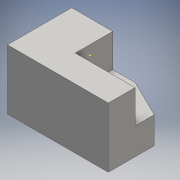
# Autodesk Inventor part: 240503_3Dsketch04
Saved by Autodesk Inventor 2016 (Build 200138000, 138)
## iProperties
Created: 2024-05-03
Part Number: 240503_3Dsketch04
Material: 일반
Document SubType Name: Modeling
Designer: pc
Density: 1 g/cm^3
Appearance: 기본값
Author: pc
Autodesk Inventor part; units mm, degrees
ref_plane "YZ Plane" through (0, 0, 0) normal (1, 0, 0) x (0, 1, 0)
ref_plane "XZ Plane" through (0, 0, 0) normal (0, 1, 0) x (-1, 0, 0)
ref_plane "XY Plane" through (0, 0, 0) normal (0, 0, 1) x (1, 0, 0)
sketch "스케치1" plane through (0, 0, 0) normal (0, 0, 1) x (1, 0, 0)
  line L0 (33.6127, -21.4008) -> (-33.6127, -21.4008)
  line L1 (-33.6127, -21.4008) -> (-33.6127, 21.4008)
  line L2 (-33.6127, 21.4008) -> (33.6127, 21.4008)
  line L3 (33.6127, 21.4008) -> (33.6127, -21.4008)
  line L4 (33.6127, -21.4008) -> (-33.6127, 21.4008) construction
  line L5 (-33.6127, -21.4008) -> (33.6127, 21.4008) construction
  point P0 (0, 0)
  constraints: 12 end point, 2 midpoint, 2 parallel, 1 horizontal, 1 perpendicular
extrude "돌출1" add sketch "스케치1" along normal blind 40
sketch "스케치2" plane through (-33.6127, 21.4008, 0) normal (0, 1, 0) x (1, 0, 0)
  line L0 (67.2253, 0) -> (67.2253, -40) projected
  line L1 (0, -40) -> (67.2253, -40) projected
  line L2 (67.2253, -17.9861) -> (27.3679, -17.9861)
  line L3 (27.3679, -17.9861) -> (27.3679, -40)
  line L4 (27.3679, -40) -> (67.2253, -40)
  line L5 (67.2253, -40) -> (67.2253, -17.9861)
  point P0 (33.6127, 0)
  constraints: 8 end point, 2 parallel, 2 point on line, 1 horizontal, 1 perpendicular
extrude "돌출2" cut sketch "스케치2" against normal blind 25
sketch "스케치3" plane through (-6.2447, 21.4008, 17.9861) normal (0, 0, 1) x (1, 0, 0)
  point P0 (6.2447, -21.4008)
sketch "스케치4" plane through (-6.2447, 21.4008, 17.9861) normal (0, 0, 1) x (1, 0, 0)
  point P0 (6.2447, -21.4008)
sketch "스케치5" plane through (-6.2447, 21.4008, 17.9861) normal (0, 0, 1) x (1, 0, 0)
  point P0 (6.2447, -21.4008)
sketch "스케치6" plane through (-33.6127, 21.4008, 0) normal (0, 1, 0) x (1, 0, 0)
  line L0 (27.3679, -17.9861) -> (67.2253, -17.9861) projected
  line L1 (0, 0) -> (67.2253, 0) projected
  line L2 (67.2253, -17.9861) -> (39.8016, -17.9861)
  line L3 (39.8016, -17.9861) -> (39.8016, 0)
  line L4 (39.8016, 0) -> (67.2253, 0)
  line L5 (67.2253, 0) -> (67.2253, -17.9861)
  point P0 (33.6127, 0)
  constraints: 8 end point, 2 parallel, 1 horizontal, 1 perpendicular, 1 point on line
sketch "스케치7" plane through (-6.2447, 21.4008, 17.9861) normal (0, 0, 1) x (1, 0, 0)
  line L0 (-27.3679, 0) -> (39.8574, 0) projected
  line L1 (14.9296, 0) -> (39.8574, -12.2366)
  line L2 (39.8574, 0) -> (39.8574, -42.8017) projected
  point P0 (6.2447, -21.4008)
  constraints: 2 end point, 2 point on line
extrude "돌출3" cut sketch "스케치7" against normal blind 20
sketch "스케치8" plane through (0, 0, 40) normal (0, 0, 1) x (1, 0, 0)
  point P0 (0, 0)
